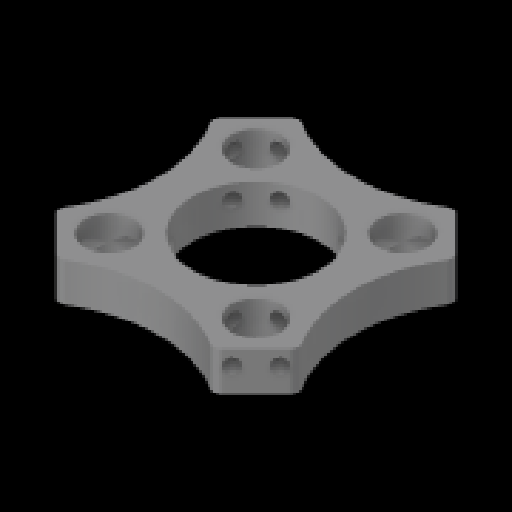
# Autodesk Inventor part: WobbleX WS12
Saved by Autodesk Inventor 2023.2 (Build 272271000, 271)
## iProperties
Created: 2023-02-17
Part Number: WobbleX WS12
Material: Aluminum 6061
Document SubType Name: Modeling
Designer: remop
Density: 2.7 g/cm^3
Appearance: Aluminum - Flat
Author: remop
Autodesk Inventor part; units mm, degrees
ref_plane "YZ Plane" through (0, 0, 0) normal (1, 0, 0) x (0, 1, 0)
ref_plane "XZ Plane" through (0, 0, 0) normal (0, 1, 0) x (-1, 0, 0)
ref_plane "XY Plane" through (0, 0, 0) normal (0, 0, 1) x (1, 0, 0)
sketch "Sketch1" plane through (0, 0, 0) normal (0, 1, 0) x (-1, 0, 0)
  circle A0 centre (0, 0) radius 13
  line L0 (-16.0122, 25) -> (-25, 16.0122)
  line L1 (-25, 16.0122) -> (-25, -16.0122) construction
  line L2 (-25, -16.0122) -> (-16.0122, -25)
  line L3 (-16.0122, -25) -> (16.0122, -25) construction
  line L4 (16.0122, -25) -> (25, -16.0122)
  line L5 (25, -16.0122) -> (25, 16.0122) construction
  line L6 (25, 16.0122) -> (16.0122, 25)
  line L7 (16.0122, 25) -> (-16.0122, 25) construction
  arc A1 (-25, -16.0122) -> (-25, 16.0122) centre (-48.139, 0) ccw
  arc A2 (-16.0122, 25) -> (16.0122, 25) centre (0, 48.139) ccw
  arc A3 (25, 16.0122) -> (25, -16.0122) centre (48.139, 0) ccw
  arc A4 (16.0122, -25) -> (-16.0122, -25) centre (0, -48.139) ccw
  circle A5 centre (-15, 15) radius 5
  circle A6 centre (15, 15) radius 5
  circle A7 centre (15, -15) radius 5
  circle A8 centre (-15, -15) radius 5
  point P0 (-25, 0)
  point P1 (25, 0)
  point P2 (0, 25)
  point P3 (0, -25)
  point P4 (0, 20)
  point P5 (0, -20)
  dimension "d0" = 26
  dimension "d3" = 5
  dimension "d4" = 30
  dimension "d5" = 30
  dimension "d6" = 15
  dimension "d7" = 15
  dimension "d8" = 10
  dimension "d12" = 58
  dimension "d13" = 40
  constraints: 16 end point, 10 point on circle, 9 centre point, 6 equal radius, 6 perpendicular, 4 horizontal alignment, 4 midpoint, 4 vertical alignment, 2 parallel, 2 vertical, 1 coincident, 1 horizontal
  measures "d0" diameter of A0
  measures "d3" distance of point (0, 20) point (0, 25)
  measures "d4" distance of A7.centre A6.centre
  measures "d5" distance of A5.centre A6.centre
  measures "d6" horizontal distance of point (0, 0) A6.centre
  measures "d7" horizontal distance of point (0, 0) A6.centre
  measures "d8" diameter of A6
  measures "d12" distance between parallel lines of L0 L4
  measures "d13" distance of point (0, 20) point (0, -20)
extrude "Extrusion1" add sketch "Sketch1" along normal blind 8
fillet "Fillet1" radius 2 8 edges at (25, 4, 16.0122) (16.0122, 4, 25) (-16.0122, 4, 25) (-25, 4, 16.0122) (-25, 4, -16.0122) (-16.0122, 4, -25) (16.0122, 4, -25) (25, 4, -16.0122)
sketch "Sketch2" plane through (17.1586, 0, 23.8536) normal (0.7071, 0, 0.7071) x (0.7071, 0, -0.7071)
  line L0 (0, 0) -> (0, 8) projected
  line L1 (0, 0) -> (9.468, 0) projected
  line L2 (9.468, 8) -> (9.468, 0) projected
  line L3 (0, 8) -> (9.468, 8) projected
  line L4 (0, 0) -> (9.468, 0) projected
  point P0 (4.734, 0)
  point P1 (1.234, 5)
  point P2 (8.234, 5)
  point P3 (4.734, 0)
  point P4 (4.734, 0)
  dimension "d14" = 3.5
  dimension "d15" = 3.5
  dimension "d16" = 5
  constraints: 2 midpoint, 1 horizontal alignment
  measures "d14" horizontal distance of point (4.734, 0) point (1.234, 5)
  measures "d15" horizontal distance of point (4.734, 0) point (8.234, 5)
  measures "d16" distance from line of L1 point (1.234, 5)
hole "Hole1" at (18.0312, 5, 22.981) at (22.981, 5, 18.0312) direction (-0.7071, 0, -0.7071) diameter 3 end through all
sketch "Sketch3" plane through (23.8536, 0, -17.1586) normal (0.7071, 0, -0.7071) x (-0.7071, 0, -0.7071)
  line L0 (0, 0) -> (0, 8) projected
  line L1 (0, 0) -> (9.468, 0) projected
  line L2 (9.468, 8) -> (9.468, 0) projected
  line L3 (0, 8) -> (9.468, 8) projected
  line L4 (0, 0) -> (9.468, 0) projected
  point P0 (4.734, 0)
  point P1 (8.234, 3)
  point P2 (1.234, 3)
  point P3 (4.734, 0)
  point P4 (4.734, 0)
  dimension "d24" = 3.5
  dimension "d25" = 5
  dimension "d26" = 3.5
  constraints: 2 midpoint, 1 horizontal alignment
  measures "d24" horizontal distance of point (8.234, 3) point (4.734, 0)
  measures "d25" distance from line of L3 point (8.234, 3)
  measures "d26" horizontal distance of point (4.734, 0) point (1.234, 3)
hole "Hole2" at (18.0312, 3, -22.981) at (22.981, 3, -18.0312) direction (-0.7071, 0, 0.7071) diameter 3 end through all
equation "\"d5\" = d4"
equation "\"d6\" = 0.5 * d5"
equation "\"d7\" = d6"
equation "\"d15\" = d14"
equation "\"d26\" = d24"
body "Solid1"
